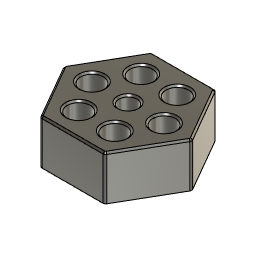
Maasi_Spin_Coater RC1 (Autodesk Fusion 360 archive; units mm, degrees)
design "Shaft_adapter_20mm"
Autodesk Fusion 360 part; units mm, degrees
sketch "Sketch1" plane through (0, 0, 0) normal (0, 0, 1) x (1, 0, 0)
  line L0 (-5.7735, 10) -> (-11.547, 0)
  line L1 (-11.547, 0) -> (-5.7735, -10)
  line L2 (-5.7735, -10) -> (5.7735, -10)
  line L3 (5.7735, -10) -> (11.547, 0)
  line L4 (11.547, 0) -> (5.7735, 10)
  line L5 (5.7735, 10) -> (-5.7735, 10)
  circle A0 centre (0, 0) radius 1.625
  circle A1 centre (-3.25, 5.6292) radius 2.05
  line L6 (0, 0) -> (-5.7735, 10) construction
  circle A2 centre (-6.5, 0) radius 2.05
  circle A3 centre (-3.25, -5.6292) radius 2.05
  circle A4 centre (3.25, -5.6292) radius 2.05
  circle A5 centre (6.5, 0) radius 2.05
  circle A6 centre (3.25, 5.6292) radius 2.05
  circle A7 centre (0, 0) radius 6.5 construction
  dimension "d1" = 10
  dimension "d2" = 3.25
  dimension "d4" = 4.1
  dimension "d9" = 360
  dimension "d10" = 13
  constraint coincident A0.centre L6.start
  constraint horizontal L5
  constraint coincident A1.centre L6
  constraint coincident A1.centre A7
  measures "d1" distance of A0.centre L5
  measures "d2" diameter of A0
  measures "d4" diameter of A1
  measures "d10" diameter of A7
extrude "Extrude1" add sketch "Sketch1" along normal blind 8
chamfer "Chamfer2" distance 0.3 angle 45 7 edges at (-8.4113, 0.7413, 8) (-5.1613, 6.3705, 8) (-1.515, 0.5876, 8) (-5.1613, -4.8879, 8) (1.3387, -4.8879, 8) (4.5887, 0.7413, 8) (1.3387, 6.3705, 8)
chamfer "Chamfer3" distance 0.5 angle 45 1 edges at (-1.515, 0.5876, 0)
fillet "Fillet1" radius 0.5 6 edges at (-5.7735, -10, 4) (5.7735, -10, 4) (11.547, 0, 4) (5.7735, 10, 4) (-5.7735, 10, 4) (-11.547, 0, 4)
chamfer "Chamfer4" distance 0.3 angle 45 12 edges at (0, -10, 8) (5.7348, -9.933, 8) (8.6603, -5, 8) (11.4697, 0, 8) (8.6603, 5, 8) (5.7348, 9.933, 8) (0, 10, 8) (-5.7348, 9.933, 8) (-8.6603, 5, 8) (-11.4697, 0, 8) (-8.6603, -5, 8) (-5.7348, -9.933, 8)
named bodies: "Shaft_adapter"

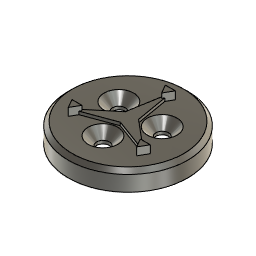
design "Round_slide_holder_20mm_param"
Autodesk Fusion 360 part; units mm, degrees
sketch "Sketch1" plane through (0, 0, 0) normal (0, 0, 1) x (1, 0, 0) in component "Round Holder  parametric"
  circle A0 centre (0, 0) radius 15.5
  line L0 (0, 11.547) -> (-10, 5.7735)
  line L1 (-10, 5.7735) -> (-10, -5.7735)
  line L2 (-10, -5.7735) -> (0, -11.547)
  line L3 (0, -11.547) -> (10, -5.7735)
  line L4 (10, -5.7735) -> (10, 5.7735)
  line L5 (10, 5.7735) -> (0, 11.547)
  line L6 (-10.3, 5.9467) -> (-10.3, -5.9467)
  line L7 (-10.3, -5.9467) -> (0, -11.8934)
  line L8 (0, -11.8934) -> (10.3, -5.9467)
  line L9 (10.3, -5.9467) -> (10.3, 5.9467)
  line L10 (10.3, 5.9467) -> (0, 11.8934)
  line L11 (0, 11.8934) -> (-10.3, 5.9467)
  circle A1 centre (0, 0) radius 10.25 construction
  line L12 (0, 8.75) -> (1.299, 11)
  line L13 (1.299, 11) -> (-1.299, 11)
  line L14 (-1.299, 11) -> (0, 8.75)
  line L15 (-1.7321, 1) -> (0, -2) construction
  line L16 (0, -2) -> (1.7321, 1) construction
  line L17 (1.7321, 1) -> (-1.7321, 1) construction
  line L18 (-1.7321, 1) -> (0, 11)
  line L19 (0, 11) -> (1.7321, 1)
  line L20 (0, -2) -> (-9.5263, -5.5)
  line L21 (-9.5263, -5.5) -> (-1.7321, 1)
  line L22 (1.7321, 1) -> (9.5263, -5.5)
  line L23 (9.5263, -5.5) -> (0, -2)
  line L24 (-7.5777, -4.375) -> (-10.1758, -4.375)
  line L25 (-10.1758, -4.375) -> (-8.8768, -6.625)
  line L26 (-8.8768, -6.625) -> (-7.5777, -4.375)
  line L27 (7.5777, -4.375) -> (8.8768, -6.625)
  line L28 (8.8768, -6.625) -> (10.1758, -4.375)
  line L29 (10.1758, -4.375) -> (7.5777, -4.375)
  line L30 (0, 0) -> (0, 11) construction
  circle A2 centre (0, 0) radius 6.5 construction
  circle A3 centre (0, 0) radius 6.5 construction
  circle A4 centre (0, -6.5) radius 1.65
  circle A5 centre (5.6292, 3.25) radius 1.65
  circle A6 centre (-5.6292, 3.25) radius 1.65
  line L31 (0, -11.8934) -> (0, -2) construction
  circle A7 centre (0, 0) radius 8.75 construction
  point P0 (0, 10.25)
  dimension "d46" = 31
  dimension "d54" = 10
  dimension "d55" = 0.3
  dimension "d72" = 1.5
  dimension "d73" = 1
  dimension "d82" = 360
  dimension "d84" = 360
  dimension "d86" = 13
  dimension "d90" = 13
  dimension "d91" = 3.3
  dimension "d93" = 360
  dimension "d109" = 17.5
  constraint coincident A0.centre A1.centre
  constraint concentric A0 A1
  constraint coincident A1 P0
  constraint parallel L13 L17
  constraint midpoint L13 L18.end
  constraint coincident L19 L16.end
  constraint coincident L20 L15.end
  constraint coincident L15.end L20
  constraint equal L22 L23
  constraint coincident L16.end L17.start
  constraint horizontal L13
  constraint coincident L12.start L30
  constraint coincident A2 A4.centre
  constraint vertical L9
  constraint coincident A4.centre L31
  constraint concentric A1 A7
  constraint coincident L12.start A7
  measures "d46" diameter of A0
  measures "d54" distance of A0.centre L5
  measures "d72" distance of L12.start P0
  measures "d73" distance of A0.centre L17
  measures "d86" diameter of A2
  measures "d90" diameter of A3
  measures "d91" diameter of A4
  measures "d109" diameter of A7
extrude "Extrude1" add sketch "Sketch1" along normal blind 5 contours A0 | L0 L5 L13 | L0 L13 L14 L18 | L0 L13 L14 | L5 L12 L13 | L5 L12 L13 L19 | L0 L1 L14 L18 L21 L24 | L12 L14 L18 L19 | L4 L5 L12 L19 L22 L29 | L12 L14 L18 L19 L20 L21 L22 L23 L24 L26 L27 L29 | L1 L21 L24 L25 | L1 L24 L25 | L4 L28 L29 | L4 L22 L28 L29 | L1 L2 L25 | L20 L21 L24 L26 | L22 L23 L27 L29 | L3 L4 L28 | L2 L20 L25 L26 | L3 L23 L27 L28 | L2 L25 L26 | L2 L3 L20 L23 L26 L27 | L3 L27 L28 | L6 L7 L8 L9 L10 L11 | A4 | A5 | A6 in component "Round Holder  parametric"
extrude "Extrude10" cut sketch "Sketch1" along normal blind 2 contours L0 L5 L13 | L0 L13 L14 L18 | L0 L13 L14 | L5 L12 L13 | L5 L12 L13 L19 | L0 L1 L14 L18 L21 L24 | L12 L14 L18 L19 | L4 L5 L12 L19 L22 L29 | L12 L14 L18 L19 L20 L21 L22 L23 L24 L26 L27 L29 | L1 L21 L24 L25 | L1 L24 L25 | L4 L28 L29 | L4 L22 L28 L29 | L1 L2 L25 | L20 L21 L24 L26 | L22 L23 L27 L29 | L3 L4 L28 | L2 L20 L25 L26 | L3 L23 L27 L28 | L2 L25 L26 | L2 L3 L20 L23 L26 L27 | L3 L27 L28 | L6 L7 L8 L9 L10 L11 | A4 | A5 | A6 in component "Round Holder  parametric"
extrude "Extrude11" add sketch "Sketch1" along normal blind 0.8 from surface at 5 contours L12 L14 L18 L19 | L12 L14 L18 L19 L20 L21 L22 L23 L24 L26 L27 L29 | L20 L21 L24 L26 | L22 L23 L27 L29 in component "Round Holder  parametric"
extrude "Extrude12" add sketch "Sketch1" along normal blind 2 from surface at 5 contours L0 L13 L14 L18 | L0 L13 L14 | L5 L12 L13 | L5 L12 L13 L19 | L12 L14 L18 L19 | L1 L21 L24 L25 | L1 L24 L25 | L4 L28 L29 | L4 L22 L28 L29 | L20 L21 L24 L26 | L22 L23 L27 L29 | L2 L20 L25 L26 | L3 L23 L27 L28 | L2 L25 L26 | L3 L27 L28 in component "Round Holder  parametric"
extrude "Extrude13" cut sketch "Sketch1" along normal through all contours A4 | A5 | A6 in component "Round Holder  parametric"
chamfer "Chamfer3" distance 2.2 angle 45 3 edges at (-1.5383, -5.9033, 5) (-7.1675, 3.8467, 5) (4.0908, 3.8467, 5) in component "Round Holder  parametric"
chamfer "Chamfer4" distance 1 angle 45 1 edges at (-14.4511, -5.605, 5) in component "Round Holder  parametric"
component "Round Holder  parametric" placed x (1, 0, 0) y (0, 1, 0) z (0, 0, 1) at (0, 0, 0)
equation "d46 = slide_diam + 13 mm"
equation "slide_diam = 18 mm"
equation "print_compensation = 0.5 mm"
equation "d109 = slide_diam - print_compensation"
named bodies: "Round_holder_18mm"

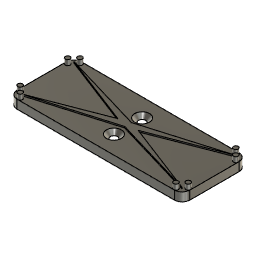
design "Square_slide_holder_20mm_param"
Autodesk Fusion 360 part; units mm, degrees
sketch "Sketch1" plane through (0, 0, 0) normal (0, 0, 1) x (1, 0, 0) in component "Square Holder parametric"
  line L0 (-10, 5.7735) -> (-10, -5.7735)
  line L1 (-10, -5.7735) -> (0, -11.547)
  line L2 (0, -11.547) -> (10, -5.7735)
  line L3 (10, -5.7735) -> (10, 5.7735)
  line L4 (10, 5.7735) -> (0, 11.547)
  line L5 (0, 11.547) -> (-10, 5.7735)
  line L6 (-10.3, -5.9467) -> (0, -11.8934)
  line L7 (0, -11.8934) -> (10.3, -5.9467)
  line L8 (10.3, -5.9467) -> (10.3, 5.9467)
  line L9 (10.3, 5.9467) -> (0, 11.8934)
  line L10 (0, 11.8934) -> (-10.3, 5.9467)
  line L11 (-10.3, 5.9467) -> (-10.3, -5.9467)
  circle A0 centre (0, 0) radius 12.5
  circle A1 centre (-35.9716, 13.8) radius 1.1
  circle A2 centre (-38.8, 10.9716) radius 1.1
  line L12 (-37.7, 12.7) -> (37.7, 12.7) construction
  line L13 (37.7, 12.7) -> (37.7, -12.7) construction
  line L14 (37.7, -12.7) -> (-37.7, -12.7) construction
  line L15 (-37.7, -12.7) -> (-37.7, 12.7) construction
  line L16 (-37.7, 12.7) -> (37.7, -12.7) construction
  line L17 (37.7, 12.7) -> (-37.7, -12.7) construction
  line L18 (-35.9716, 13.8) -> (-38.8, 10.9716) construction
  line L19 (39.9, -14.9) -> (-39.9, -14.9)
  line L20 (-39.9, -14.9) -> (-39.9, 14.9)
  line L21 (-39.9, 14.9) -> (39.9, 14.9)
  line L22 (39.9, 14.9) -> (39.9, -14.9)
  line L23 (-38.8, 10.9716) -> (-39.9, 14.9) construction
  line L24 (-35.9716, 13.8) -> (-39.9, 14.9) construction
  line L25 (1.75, 0) -> (22.5, 0) construction
  circle A3 centre (-35.9716, -13.8) radius 1.1
  circle A4 centre (-38.8, -10.9716) radius 1.1
  line L26 (0, 1.75) -> (0, 22.5) construction
  circle A5 centre (35.9716, 13.8) radius 1.1
  circle A6 centre (35.9716, -13.8) radius 1.1
  circle A7 centre (38.8, -10.9716) radius 1.1
  circle A8 centre (38.8, 10.9716) radius 1.1
  line L27 (-37.7, 12.7) -> (-4.7125, 0)
  line L28 (-4.7125, 0) -> (-37.7, -12.7)
  line L29 (-37.7, 12.7) -> (0, 1.5625)
  line L30 (-37.7, -12.7) -> (0, -1.5625)
  line L31 (37.7, 12.7) -> (0, 1.5625)
  line L32 (37.7, 12.7) -> (4.7125, 0)
  line L33 (4.7125, 0) -> (37.7, -12.7)
  line L34 (37.7, -12.7) -> (0, -1.5625)
  circle A9 centre (0, 0) radius 6.5 construction
  line L35 (0, 0) -> (0, -11.8934) construction
  circle A10 centre (0, -6.5) radius 1.65
  circle A11 centre (0, 6.5) radius 1.65
  dimension "d92" = 10
  dimension "d93" = 0.3
  dimension "d94" = 25
  dimension "d101" = 4
  dimension "d103" = -2.2
  dimension "d104" = 75.4
  dimension "d105" = 25.4
  dimension "d115" = 9.425
  dimension "d116" = 3.125
  dimension "d123" = 13
  dimension "d124" = 3.3
  constraint coincident A0.centre A9.centre
  constraint equal A1 A2
  constraint horizontal L12
  constraint perpendicular L12 L13
  constraint parallel L12 L14
  constraint parallel L13 L15
  constraint coincident L16 A0.centre
  constraint coincident L17 A0.centre
  constraint tangent A1 L12
  constraint tangent A2 L15
  constraint coincident A1.centre L18.start
  constraint coincident A2.centre L18.end
  constraint tangent A1 L21
  constraint equal L23 L24
  constraint symmetric A1 L25 A3
  constraint symmetric A2 L25 A4
  constraint symmetric A1 L26 A5
  constraint symmetric A2 L26 A8
  constraint symmetric A3 L26 A6
  constraint symmetric A4 L26 A7
  constraint coincident L26 L29.end
  constraint symmetric L25 L29 L30
  constraint symmetric L25 L27 L28
  constraint symmetric L12.start L26 L12.end
  constraint symmetric L14.end L26 L13.end
  constraint symmetric L26 L27.end L32.end
  constraint symmetric L26 L29.end L31.end
  constraint symmetric L26 L30.end L34.end
  constraint coincident L30.end L34.end
  constraint vertical L8
  constraint coincident A9 A10.centre
  constraint coincident L35 A10.centre
  constraint symmetric L25 A10 A11
  measures "d92" distance of A0.centre L5
  measures "d94" diameter of A0
  measures "d101" distance of A1.centre A2.centre
  measures "d104" distance of L12.start L12.end
  measures "d105" distance of L12.end L13.end
  measures "d115" distance of L27.end L32.end
  measures "d116" distance of L29.end L30.end
  measures "d123" diameter of A9
  measures "d124" diameter of A10
extrude "Extrude9" add sketch "Sketch1" along normal blind 4 contours L0 L3 L4 L5 L29 L31 | L0 L3 L4 L5 L8 L9 L10 L11 L29 L31 | L0 L3 L27 L28 L29 L30 L31 L32 L33 L34 | L0 L11 L27 L29 | L0 L27 L28 | L0 L11 L27 L28 | L8 L9 L10 L11 A0 L29 L31 | L11 A0 L27 L29 | L0 L11 L28 L30 | L11 A0 L27 L28 | A0 L27 L29 | L3 L8 L31 L32 | L0 L1 L2 L3 L30 L34 | L0 L1 L2 L3 L6 L7 L8 L11 L30 L34 | L11 A0 L28 L30 | A0 L31 L32 | L8 A0 L31 L32 | L3 L8 L32 L33 | L3 L32 L33 | L6 L7 L8 L11 A0 L30 L34 | A0 L28 L30 | L8 A0 L32 L33 | L3 L8 L33 L34 | L8 A0 L33 L34 | A0 L33 L34 | A1 | A2 | A4 | A3 | A6 | A7 | A8 | A5 | L19 L20 L21 L22 | A10 | A11 in component "Square Holder parametric"
extrude "Extrude11" add sketch "Sketch1" along normal blind 2.4 from surface at 4 contours A1 | A2 | A4 | A3 | A6 | A7 | A8 | A5 in component "Square Holder parametric"
extrude "Extrude13" cut sketch "Sketch1" along normal blind 2.2 contours L0 L3 L4 L5 L29 L31 | L0 L3 L4 L5 L8 L9 L10 L11 L29 L31 | L0 L3 L27 L28 L29 L30 L31 L32 L33 L34 | L0 L11 L27 L29 | L0 L27 L28 | L0 L11 L27 L28 | L0 L11 L28 L30 | L3 L8 L31 L32 | L0 L1 L2 L3 L30 L34 | L0 L1 L2 L3 L6 L7 L8 L11 L30 L34 | L3 L8 L32 L33 | L3 L32 L33 | L3 L8 L33 L34 | A10 | A11 in component "Square Holder parametric"
extrude "Extrude12" add sketch "Sketch1" along normal blind 0.6 from surface at 4 contours L0 L3 L27 L28 L29 L30 L31 L32 L33 L34 | L0 L11 L27 L29 | L11 A0 L27 L29 | L0 L11 L28 L30 | A0 L27 L29 | L3 L8 L31 L32 | L11 A0 L28 L30 | A0 L31 L32 | L8 A0 L31 L32 | A0 L28 L30 | L3 L8 L33 L34 | L8 A0 L33 L34 | A0 L33 L34 in component "Square Holder parametric"
extrude "Extrude14" cut sketch "Sketch1" along normal through all contours A10 | A11 in component "Square Holder parametric"
chamfer "Chamfer2" distance 1.8 angle 45 2 edges at (-1.5383, -5.9033, 4) (-1.5383, 7.0967, 4) in component "Square Holder parametric"
fillet "Fillet1" radius 3.5 4 edges at (39.9, 14.9, 2) (-39.9, 14.9, 2) (-39.9, -14.9, 2) (39.9, -14.9, 2) in component "Square Holder parametric"
component "Square Holder parametric" placed x (1, 0, 0) y (0, 1, 0) z (0, 0, 1) at (0, 0, 0)
equation "slide_height = 25 mm"
equation "print_compensation = 0.2 mm"
equation "d104 = slide_width + 0.4 mm"
equation "d105 = slide_height + 0.4 mm"
equation "d115 = d104 / 8"
equation "d116 = slide_height / 8"
equation "slide_width = 75 mm"
named bodies: "Square_holder_75x25"
